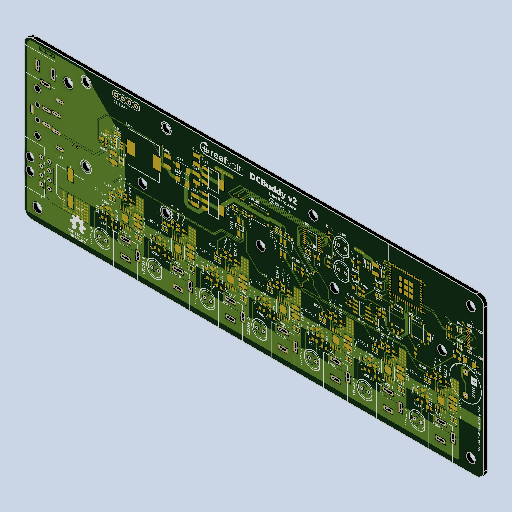
# Autodesk Inventor part: dcbuddy_v2_BOARD
Saved by Autodesk Inventor 2024.3 (Build 283343000, 343)
## iProperties
Created: 2024-05-05
Part Number: dcbuddy_v2_BOARD
Material: Generic
Document SubType Name: Modeling
Designer: atrus
Density: 1 g/cm^3
Appearance: BoardColor
Author: atrus
Autodesk Inventor part; units mm, degrees
ref_plane "YZ Plane" through (0, 0, 0) normal (1, 0, 0) x (0, 1, 0)
ref_plane "XZ Plane" through (0, 0, 0) normal (0, 1, 0) x (-1, 0, 0)
ref_plane "BoardFrontPlane" through (0, 0, 0) normal (0, 0, 1) x (1, 0, 0)
sketch "Sketch1" plane through (0, 0, 0) normal (0, 0, 1) x (1, 0, 0)
  arc A0 (36, 33) -> (39, 30) centre (39, 33) ccw
  line L0 (39, 30) -> (208, 30)
  arc A1 (208, 30) -> (211, 33) centre (208, 33) ccw
  line L1 (211, 33) -> (211, 87)
  arc A2 (211, 87) -> (208, 90) centre (208, 87) ccw
  line L2 (208, 90) -> (39, 90)
  arc A3 (39, 90) -> (36, 87) centre (39, 87) ccw
  line L3 (36, 87) -> (36, 33)
  constraints: 8 end point, 8 point on circle, 4 centre point
extrude "BoardOutline" add sketch "Sketch1" along normal blind 1.4202
sketch "Sketch19" plane through (0, 0, 1.4202) normal (0, 0, 1) x (1, 0, 0)
  point P0 (158.24, 80)
hole "LED301-C" at (158.24, 80, 1.4202) direction (0, 0, -1) diameter 0.8128 end through all
sketch "Sketch20" plane through (0, 0, 1.4202) normal (0, 0, 1) x (1, 0, 0)
  point P0 (155.7, 80)
hole "LED301-A" at (155.7, 80, 1.4202) direction (0, 0, -1) diameter 0.8128 end through all
sketch "Sketch21" plane through (0, 0, 1.4202) normal (0, 0, 1) x (1, 0, 0)
  point P0 (158.24, 72)
hole "LED300-C" at (158.24, 72, 1.4202) direction (0, 0, -1) diameter 0.8128 end through all
sketch "Sketch22" plane through (0, 0, 1.4202) normal (0, 0, 1) x (1, 0, 0)
  point P0 (155.7, 72)
hole "LED300-A" at (155.7, 72, 1.4202) direction (0, 0, -1) diameter 0.8128 end through all
sketch "Sketch23" plane through (0, 0, 1.4202) normal (0, 0, 1) x (1, 0, 0)
  point P0 (187.04, 37.25)
hole "LED200_CH7-C" at (187.04, 37.25, 1.4202) direction (0, 0, -1) diameter 0.8128 end through all
sketch "Sketch24" plane through (0, 0, 1.4202) normal (0, 0, 1) x (1, 0, 0)
  point P0 (184.5, 37.25)
hole "LED200_CH7-A" at (184.5, 37.25, 1.4202) direction (0, 0, -1) diameter 0.8128 end through all
sketch "Sketch25" plane through (0, 0, 1.4202) normal (0, 0, 1) x (1, 0, 0)
  point P0 (167.04, 37.25)
hole "LED200_CH6-C" at (167.04, 37.25, 1.4202) direction (0, 0, -1) diameter 0.8128 end through all
sketch "Sketch26" plane through (0, 0, 1.4202) normal (0, 0, 1) x (1, 0, 0)
  point P0 (164.5, 37.25)
hole "LED200_CH6-A" at (164.5, 37.25, 1.4202) direction (0, 0, -1) diameter 0.8128 end through all
sketch "Sketch27" plane through (0, 0, 1.4202) normal (0, 0, 1) x (1, 0, 0)
  point P0 (147.04, 37.25)
hole "LED200_CH5-C" at (147.04, 37.25, 1.4202) direction (0, 0, -1) diameter 0.8128 end through all
sketch "Sketch28" plane through (0, 0, 1.4202) normal (0, 0, 1) x (1, 0, 0)
  point P0 (144.5, 37.25)
hole "LED200_CH5-A" at (144.5, 37.25, 1.4202) direction (0, 0, -1) diameter 0.8128 end through all
sketch "Sketch29" plane through (0, 0, 1.4202) normal (0, 0, 1) x (1, 0, 0)
  point P0 (127.04, 37.25)
hole "LED200_CH4-C" at (127.04, 37.25, 1.4202) direction (0, 0, -1) diameter 0.8128 end through all
sketch "Sketch30" plane through (0, 0, 1.4202) normal (0, 0, 1) x (1, 0, 0)
  point P0 (124.5, 37.25)
hole "LED200_CH4-A" at (124.5, 37.25, 1.4202) direction (0, 0, -1) diameter 0.8128 end through all
sketch "Sketch31" plane through (0, 0, 1.4202) normal (0, 0, 1) x (1, 0, 0)
  point P0 (107.04, 37.25)
hole "LED200_CH3-C" at (107.04, 37.25, 1.4202) direction (0, 0, -1) diameter 0.8128 end through all
sketch "Sketch32" plane through (0, 0, 1.4202) normal (0, 0, 1) x (1, 0, 0)
  point P0 (104.5, 37.25)
hole "LED200_CH3-A" at (104.5, 37.25, 1.4202) direction (0, 0, -1) diameter 0.8128 end through all
sketch "Sketch33" plane through (0, 0, 1.4202) normal (0, 0, 1) x (1, 0, 0)
  point P0 (87.04, 37.25)
hole "LED200_CH2-C" at (87.04, 37.25, 1.4202) direction (0, 0, -1) diameter 0.8128 end through all
sketch "Sketch34" plane through (0, 0, 1.4202) normal (0, 0, 1) x (1, 0, 0)
  point P0 (84.5, 37.25)
hole "LED200_CH2-A" at (84.5, 37.25, 1.4202) direction (0, 0, -1) diameter 0.8128 end through all
sketch "Sketch35" plane through (0, 0, 1.4202) normal (0, 0, 1) x (1, 0, 0)
  point P0 (67.04, 37.25)
hole "LED200_CH1-C" at (67.04, 37.25, 1.4202) direction (0, 0, -1) diameter 0.8128 end through all
sketch "Sketch36" plane through (0, 0, 1.4202) normal (0, 0, 1) x (1, 0, 0)
  point P0 (64.5, 37.25)
hole "LED200_CH1-A" at (64.5, 37.25, 1.4202) direction (0, 0, -1) diameter 0.8128 end through all
sketch "Sketch37" plane through (0, 0, 1.4202) normal (0, 0, 1) x (1, 0, 0)
  line L0 (45, 77.3) -> (43, 77.3) construction
  line L1 (45, 77.8) -> (43, 77.8)
  line L2 (43, 76.8) -> (45, 76.8)
  arc A0 (45, 76.8) -> (45, 77.8) centre (45, 77.3) ccw
  arc A1 (43, 77.8) -> (43, 76.8) centre (43, 77.3) ccw
  point P0 (44, 77.3)
  constraints: 8 end point, 4 point on circle, 4 tangent, 2 centre point, 1 midpoint, 1 parallel
extrude "J701-3" cut sketch "Sketch37" against normal through all
sketch "Sketch38" plane through (0, 0, 1.4202) normal (0, 0, 1) x (1, 0, 0)
  line L0 (41, 81) -> (41, 83) construction
  line L1 (41.5, 81) -> (41.5, 83)
  line L2 (40.5, 83) -> (40.5, 81)
  arc A0 (40.5, 81) -> (41.5, 81) centre (41, 81) ccw
  arc A1 (41.5, 83) -> (40.5, 83) centre (41, 83) ccw
  point P0 (41, 82)
  constraints: 8 end point, 4 point on circle, 4 tangent, 2 centre point, 1 midpoint, 1 parallel
extrude "J701-2" cut sketch "Sketch38" against normal through all
sketch "Sketch39" plane through (0, 0, 1.4202) normal (0, 0, 1) x (1, 0, 0)
  line L0 (47, 80.75) -> (47, 83.25) construction
  line L1 (47.5, 80.75) -> (47.5, 83.25)
  line L2 (46.5, 83.25) -> (46.5, 80.75)
  arc A0 (46.5, 80.75) -> (47.5, 80.75) centre (47, 80.75) ccw
  arc A1 (47.5, 83.25) -> (46.5, 83.25) centre (47, 83.25) ccw
  point P0 (47, 82)
  constraints: 8 end point, 4 point on circle, 4 tangent, 2 centre point, 1 midpoint, 1 parallel
extrude "J701-1" cut sketch "Sketch39" against normal through all
sketch "Sketch40" plane through (0, 0, 1.4202) normal (0, 0, 1) x (1, 0, 0)
  line L0 (199.2, 39.25) -> (199.2, 37.25) construction
  line L1 (198.7, 39.25) -> (198.7, 37.25)
  line L2 (199.7, 37.25) -> (199.7, 39.25)
  arc A0 (199.7, 39.25) -> (198.7, 39.25) centre (199.2, 39.25) ccw
  arc A1 (198.7, 37.25) -> (199.7, 37.25) centre (199.2, 37.25) ccw
  point P0 (199.2, 38.25)
  constraints: 8 end point, 4 point on circle, 4 tangent, 2 centre point, 1 midpoint, 1 parallel
extrude "J200_CH7-3" cut sketch "Sketch40" against normal through all
sketch "Sketch41" plane through (0, 0, 1.4202) normal (0, 0, 1) x (1, 0, 0)
  line L0 (195.5, 35.25) -> (193.5, 35.25) construction
  line L1 (195.5, 35.75) -> (193.5, 35.75)
  line L2 (193.5, 34.75) -> (195.5, 34.75)
  arc A0 (195.5, 34.75) -> (195.5, 35.75) centre (195.5, 35.25) ccw
  arc A1 (193.5, 35.75) -> (193.5, 34.75) centre (193.5, 35.25) ccw
  point P0 (194.5, 35.25)
  constraints: 8 end point, 4 point on circle, 4 tangent, 2 centre point, 1 midpoint, 1 parallel
extrude "J200_CH7-2" cut sketch "Sketch41" against normal through all
sketch "Sketch42" plane through (0, 0, 1.4202) normal (0, 0, 1) x (1, 0, 0)
  line L0 (195.75, 41.25) -> (193.25, 41.25) construction
  line L1 (195.75, 41.75) -> (193.25, 41.75)
  line L2 (193.25, 40.75) -> (195.75, 40.75)
  arc A0 (195.75, 40.75) -> (195.75, 41.75) centre (195.75, 41.25) ccw
  arc A1 (193.25, 41.75) -> (193.25, 40.75) centre (193.25, 41.25) ccw
  point P0 (194.5, 41.25)
  constraints: 8 end point, 4 point on circle, 4 tangent, 2 centre point, 1 midpoint, 1 parallel
extrude "J200_CH7-1" cut sketch "Sketch42" against normal through all
sketch "Sketch43" plane through (0, 0, 1.4202) normal (0, 0, 1) x (1, 0, 0)
  line L0 (179.2, 39.25) -> (179.2, 37.25) construction
  line L1 (178.7, 39.25) -> (178.7, 37.25)
  line L2 (179.7, 37.25) -> (179.7, 39.25)
  arc A0 (179.7, 39.25) -> (178.7, 39.25) centre (179.2, 39.25) ccw
  arc A1 (178.7, 37.25) -> (179.7, 37.25) centre (179.2, 37.25) ccw
  point P0 (179.2, 38.25)
  constraints: 8 end point, 4 point on circle, 4 tangent, 2 centre point, 1 midpoint, 1 parallel
extrude "J200_CH6-3" cut sketch "Sketch43" against normal through all
sketch "Sketch44" plane through (0, 0, 1.4202) normal (0, 0, 1) x (1, 0, 0)
  line L0 (175.5, 35.25) -> (173.5, 35.25) construction
  line L1 (175.5, 35.75) -> (173.5, 35.75)
  line L2 (173.5, 34.75) -> (175.5, 34.75)
  arc A0 (175.5, 34.75) -> (175.5, 35.75) centre (175.5, 35.25) ccw
  arc A1 (173.5, 35.75) -> (173.5, 34.75) centre (173.5, 35.25) ccw
  point P0 (174.5, 35.25)
  constraints: 8 end point, 4 point on circle, 4 tangent, 2 centre point, 1 midpoint, 1 parallel
extrude "J200_CH6-2" cut sketch "Sketch44" against normal through all
sketch "Sketch45" plane through (0, 0, 1.4202) normal (0, 0, 1) x (1, 0, 0)
  line L0 (175.75, 41.25) -> (173.25, 41.25) construction
  line L1 (175.75, 41.75) -> (173.25, 41.75)
  line L2 (173.25, 40.75) -> (175.75, 40.75)
  arc A0 (175.75, 40.75) -> (175.75, 41.75) centre (175.75, 41.25) ccw
  arc A1 (173.25, 41.75) -> (173.25, 40.75) centre (173.25, 41.25) ccw
  point P0 (174.5, 41.25)
  constraints: 8 end point, 4 point on circle, 4 tangent, 2 centre point, 1 midpoint, 1 parallel
extrude "J200_CH6-1" cut sketch "Sketch45" against normal through all
sketch "Sketch46" plane through (0, 0, 1.4202) normal (0, 0, 1) x (1, 0, 0)
  line L0 (159.2, 39.25) -> (159.2, 37.25) construction
  line L1 (158.7, 39.25) -> (158.7, 37.25)
  line L2 (159.7, 37.25) -> (159.7, 39.25)
  arc A0 (159.7, 39.25) -> (158.7, 39.25) centre (159.2, 39.25) ccw
  arc A1 (158.7, 37.25) -> (159.7, 37.25) centre (159.2, 37.25) ccw
  point P0 (159.2, 38.25)
  constraints: 8 end point, 4 point on circle, 4 tangent, 2 centre point, 1 midpoint, 1 parallel
extrude "J200_CH5-3" cut sketch "Sketch46" against normal through all
sketch "Sketch47" plane through (0, 0, 1.4202) normal (0, 0, 1) x (1, 0, 0)
  line L0 (155.5, 35.25) -> (153.5, 35.25) construction
  line L1 (155.5, 35.75) -> (153.5, 35.75)
  line L2 (153.5, 34.75) -> (155.5, 34.75)
  arc A0 (155.5, 34.75) -> (155.5, 35.75) centre (155.5, 35.25) ccw
  arc A1 (153.5, 35.75) -> (153.5, 34.75) centre (153.5, 35.25) ccw
  point P0 (154.5, 35.25)
  constraints: 8 end point, 4 point on circle, 4 tangent, 2 centre point, 1 midpoint, 1 parallel
extrude "J200_CH5-2" cut sketch "Sketch47" against normal through all
sketch "Sketch48" plane through (0, 0, 1.4202) normal (0, 0, 1) x (1, 0, 0)
  line L0 (155.75, 41.25) -> (153.25, 41.25) construction
  line L1 (155.75, 41.75) -> (153.25, 41.75)
  line L2 (153.25, 40.75) -> (155.75, 40.75)
  arc A0 (155.75, 40.75) -> (155.75, 41.75) centre (155.75, 41.25) ccw
  arc A1 (153.25, 41.75) -> (153.25, 40.75) centre (153.25, 41.25) ccw
  point P0 (154.5, 41.25)
  constraints: 8 end point, 4 point on circle, 4 tangent, 2 centre point, 1 midpoint, 1 parallel
extrude "J200_CH5-1" cut sketch "Sketch48" against normal through all
sketch "Sketch49" plane through (0, 0, 1.4202) normal (0, 0, 1) x (1, 0, 0)
  line L0 (139.2, 39.25) -> (139.2, 37.25) construction
  line L1 (138.7, 39.25) -> (138.7, 37.25)
  line L2 (139.7, 37.25) -> (139.7, 39.25)
  arc A0 (139.7, 39.25) -> (138.7, 39.25) centre (139.2, 39.25) ccw
  arc A1 (138.7, 37.25) -> (139.7, 37.25) centre (139.2, 37.25) ccw
  point P0 (139.2, 38.25)
  constraints: 8 end point, 4 point on circle, 4 tangent, 2 centre point, 1 midpoint, 1 parallel
extrude "J200_CH4-3" cut sketch "Sketch49" against normal through all
sketch "Sketch50" plane through (0, 0, 1.4202) normal (0, 0, 1) x (1, 0, 0)
  line L0 (135.5, 35.25) -> (133.5, 35.25) construction
  line L1 (135.5, 35.75) -> (133.5, 35.75)
  line L2 (133.5, 34.75) -> (135.5, 34.75)
  arc A0 (135.5, 34.75) -> (135.5, 35.75) centre (135.5, 35.25) ccw
  arc A1 (133.5, 35.75) -> (133.5, 34.75) centre (133.5, 35.25) ccw
  point P0 (134.5, 35.25)
  constraints: 8 end point, 4 point on circle, 4 tangent, 2 centre point, 1 midpoint, 1 parallel
extrude "J200_CH4-2" cut sketch "Sketch50" against normal through all
sketch "Sketch51" plane through (0, 0, 1.4202) normal (0, 0, 1) x (1, 0, 0)
  line L0 (135.75, 41.25) -> (133.25, 41.25) construction
  line L1 (135.75, 41.75) -> (133.25, 41.75)
  line L2 (133.25, 40.75) -> (135.75, 40.75)
  arc A0 (135.75, 40.75) -> (135.75, 41.75) centre (135.75, 41.25) ccw
  arc A1 (133.25, 41.75) -> (133.25, 40.75) centre (133.25, 41.25) ccw
  point P0 (134.5, 41.25)
  constraints: 8 end point, 4 point on circle, 4 tangent, 2 centre point, 1 midpoint, 1 parallel
extrude "J200_CH4-1" cut sketch "Sketch51" against normal through all
sketch "Sketch52" plane through (0, 0, 1.4202) normal (0, 0, 1) x (1, 0, 0)
  line L0 (119.2, 39.25) -> (119.2, 37.25) construction
  line L1 (118.7, 39.25) -> (118.7, 37.25)
  line L2 (119.7, 37.25) -> (119.7, 39.25)
  arc A0 (119.7, 39.25) -> (118.7, 39.25) centre (119.2, 39.25) ccw
  arc A1 (118.7, 37.25) -> (119.7, 37.25) centre (119.2, 37.25) ccw
  point P0 (119.2, 38.25)
  constraints: 8 end point, 4 point on circle, 4 tangent, 2 centre point, 1 midpoint, 1 parallel
extrude "J200_CH3-3" cut sketch "Sketch52" against normal through all
sketch "Sketch53" plane through (0, 0, 1.4202) normal (0, 0, 1) x (1, 0, 0)
  line L0 (115.5, 35.25) -> (113.5, 35.25) construction
  line L1 (115.5, 35.75) -> (113.5, 35.75)
  line L2 (113.5, 34.75) -> (115.5, 34.75)
  arc A0 (115.5, 34.75) -> (115.5, 35.75) centre (115.5, 35.25) ccw
  arc A1 (113.5, 35.75) -> (113.5, 34.75) centre (113.5, 35.25) ccw
  point P0 (114.5, 35.25)
  constraints: 8 end point, 4 point on circle, 4 tangent, 2 centre point, 1 midpoint, 1 parallel
extrude "J200_CH3-2" cut sketch "Sketch53" against normal through all
sketch "Sketch54" plane through (0, 0, 1.4202) normal (0, 0, 1) x (1, 0, 0)
  line L0 (115.75, 41.25) -> (113.25, 41.25) construction
  line L1 (115.75, 41.75) -> (113.25, 41.75)
  line L2 (113.25, 40.75) -> (115.75, 40.75)
  arc A0 (115.75, 40.75) -> (115.75, 41.75) centre (115.75, 41.25) ccw
  arc A1 (113.25, 41.75) -> (113.25, 40.75) centre (113.25, 41.25) ccw
  point P0 (114.5, 41.25)
  constraints: 8 end point, 4 point on circle, 4 tangent, 2 centre point, 1 midpoint, 1 parallel
extrude "J200_CH3-1" cut sketch "Sketch54" against normal through all
sketch "Sketch55" plane through (0, 0, 1.4202) normal (0, 0, 1) x (1, 0, 0)
  line L0 (99.2, 39.25) -> (99.2, 37.25) construction
  line L1 (98.7, 39.25) -> (98.7, 37.25)
  line L2 (99.7, 37.25) -> (99.7, 39.25)
  arc A0 (99.7, 39.25) -> (98.7, 39.25) centre (99.2, 39.25) ccw
  arc A1 (98.7, 37.25) -> (99.7, 37.25) centre (99.2, 37.25) ccw
  point P0 (99.2, 38.25)
  constraints: 8 end point, 4 point on circle, 4 tangent, 2 centre point, 1 midpoint, 1 parallel
extrude "J200_CH2-3" cut sketch "Sketch55" against normal through all
sketch "Sketch56" plane through (0, 0, 1.4202) normal (0, 0, 1) x (1, 0, 0)
  line L0 (95.5, 35.25) -> (93.5, 35.25) construction
  line L1 (95.5, 35.75) -> (93.5, 35.75)
  line L2 (93.5, 34.75) -> (95.5, 34.75)
  arc A0 (95.5, 34.75) -> (95.5, 35.75) centre (95.5, 35.25) ccw
  arc A1 (93.5, 35.75) -> (93.5, 34.75) centre (93.5, 35.25) ccw
  point P0 (94.5, 35.25)
  constraints: 8 end point, 4 point on circle, 4 tangent, 2 centre point, 1 midpoint, 1 parallel
extrude "J200_CH2-2" cut sketch "Sketch56" against normal through all
sketch "Sketch57" plane through (0, 0, 1.4202) normal (0, 0, 1) x (1, 0, 0)
  line L0 (95.75, 41.25) -> (93.25, 41.25) construction
  line L1 (95.75, 41.75) -> (93.25, 41.75)
  line L2 (93.25, 40.75) -> (95.75, 40.75)
  arc A0 (95.75, 40.75) -> (95.75, 41.75) centre (95.75, 41.25) ccw
  arc A1 (93.25, 41.75) -> (93.25, 40.75) centre (93.25, 41.25) ccw
  point P0 (94.5, 41.25)
  constraints: 8 end point, 4 point on circle, 4 tangent, 2 centre point, 1 midpoint, 1 parallel
extrude "J200_CH2-1" cut sketch "Sketch57" against normal through all
sketch "Sketch58" plane through (0, 0, 1.4202) normal (0, 0, 1) x (1, 0, 0)
  line L0 (79.2, 39.25) -> (79.2, 37.25) construction
  line L1 (78.7, 39.25) -> (78.7, 37.25)
  line L2 (79.7, 37.25) -> (79.7, 39.25)
  arc A0 (79.7, 39.25) -> (78.7, 39.25) centre (79.2, 39.25) ccw
  arc A1 (78.7, 37.25) -> (79.7, 37.25) centre (79.2, 37.25) ccw
  point P0 (79.2, 38.25)
  constraints: 8 end point, 4 point on circle, 4 tangent, 2 centre point, 1 midpoint, 1 parallel
extrude "J200_CH1-3" cut sketch "Sketch58" against normal through all
sketch "Sketch59" plane through (0, 0, 1.4202) normal (0, 0, 1) x (1, 0, 0)
  line L0 (75.5, 35.25) -> (73.5, 35.25) construction
  line L1 (75.5, 35.75) -> (73.5, 35.75)
  line L2 (73.5, 34.75) -> (75.5, 34.75)
  arc A0 (75.5, 34.75) -> (75.5, 35.75) centre (75.5, 35.25) ccw
  arc A1 (73.5, 35.75) -> (73.5, 34.75) centre (73.5, 35.25) ccw
  point P0 (74.5, 35.25)
  constraints: 8 end point, 4 point on circle, 4 tangent, 2 centre point, 1 midpoint, 1 parallel
extrude "J200_CH1-2" cut sketch "Sketch59" against normal through all
sketch "Sketch60" plane through (0, 0, 1.4202) normal (0, 0, 1) x (1, 0, 0)
  line L0 (75.75, 41.25) -> (73.25, 41.25) construction
  line L1 (75.75, 41.75) -> (73.25, 41.75)
  line L2 (73.25, 40.75) -> (75.75, 40.75)
  arc A0 (75.75, 40.75) -> (75.75, 41.75) centre (75.75, 41.25) ccw
  arc A1 (73.25, 41.75) -> (73.25, 40.75) centre (73.25, 41.25) ccw
  point P0 (74.5, 41.25)
  constraints: 8 end point, 4 point on circle, 4 tangent, 2 centre point, 1 midpoint, 1 parallel
extrude "J200_CH1-1" cut sketch "Sketch60" against normal through all
sketch "Sketch61" plane through (0, 0, 1.4202) normal (0, 0, 1) x (1, 0, 0)
  point P0 (41, 58.7)
hole "J700-_DVCFIAIY" at (41, 58.7, 1.4202) direction (0, 0, -1) diameter 2.2 end through all
sketch "Sketch62" plane through (0, 0, 1.4202) normal (0, 0, 1) x (1, 0, 0)
  point P0 (41, 74.3)
hole "J700-_ODLUWIDP" at (41, 74.3, 1.4202) direction (0, 0, -1) diameter 2.2 end through all
sketch "Sketch63" plane through (0, 0, 1.4202) normal (0, 0, 1) x (1, 0, 0)
  line L0 (49.1, 69.4) -> (47.2, 69.4) construction
  line L1 (49.1, 69.7) -> (47.2, 69.7)
  line L2 (47.2, 69.1) -> (49.1, 69.1)
  arc A0 (49.1, 69.1) -> (49.1, 69.7) centre (49.1, 69.4) ccw
  arc A1 (47.2, 69.7) -> (47.2, 69.1) centre (47.2, 69.4) ccw
  point P0 (48.15, 69.4)
  constraints: 8 end point, 4 point on circle, 4 tangent, 2 centre point, 1 midpoint, 1 parallel
extrude "J700-1" cut sketch "Sketch63" against normal through all
sketch "Sketch64" plane through (0, 0, 1.4202) normal (0, 0, 1) x (1, 0, 0)
  line L0 (49.1, 63.6) -> (47.2, 63.6) construction
  line L1 (49.1, 63.9) -> (47.2, 63.9)
  line L2 (47.2, 63.3) -> (49.1, 63.3)
  arc A0 (49.1, 63.3) -> (49.1, 63.9) centre (49.1, 63.6) ccw
  arc A1 (47.2, 63.9) -> (47.2, 63.3) centre (47.2, 63.6) ccw
  point P0 (48.15, 63.6)
  constraints: 8 end point, 4 point on circle, 4 tangent, 2 centre point, 1 midpoint, 1 parallel
extrude "J700-2" cut sketch "Sketch64" against normal through all
sketch "Sketch65" plane through (0, 0, 1.4202) normal (0, 0, 1) x (1, 0, 0)
  line L0 (45.45, 69) -> (43.55, 69) construction
  line L1 (45.45, 69.3) -> (43.55, 69.3)
  line L2 (43.55, 68.7) -> (45.45, 68.7)
  arc A0 (45.45, 68.7) -> (45.45, 69.3) centre (45.45, 69) ccw
  arc A1 (43.55, 69.3) -> (43.55, 68.7) centre (43.55, 69) ccw
  point P0 (44.5, 69)
  constraints: 8 end point, 4 point on circle, 4 tangent, 2 centre point, 1 midpoint, 1 parallel
extrude "J700-3" cut sketch "Sketch65" against normal through all
sketch "Sketch66" plane through (0, 0, 1.4202) normal (0, 0, 1) x (1, 0, 0)
  line L0 (45.45, 64) -> (43.55, 64) construction
  line L1 (45.45, 64.3) -> (43.55, 64.3)
  line L2 (43.55, 63.7) -> (45.45, 63.7)
  arc A0 (45.45, 63.7) -> (45.45, 64.3) centre (45.45, 64) ccw
  arc A1 (43.55, 64.3) -> (43.55, 63.7) centre (43.55, 64) ccw
  point P0 (44.5, 64)
  constraints: 8 end point, 4 point on circle, 4 tangent, 2 centre point, 1 midpoint, 1 parallel
extrude "J700-4" cut sketch "Sketch66" against normal through all
sketch "Sketch67" plane through (0, 0, 1.4202) normal (0, 0, 1) x (1, 0, 0)
  line L0 (39, 65.7) -> (39, 67.3) construction
  line L1 (39.3, 65.7) -> (39.3, 67.3)
  line L2 (38.7, 67.3) -> (38.7, 65.7)
  arc A0 (38.7, 65.7) -> (39.3, 65.7) centre (39, 65.7) ccw
  arc A1 (39.3, 67.3) -> (38.7, 67.3) centre (39, 67.3) ccw
  point P0 (39, 66.5)
  constraints: 8 end point, 4 point on circle, 4 tangent, 2 centre point, 1 midpoint, 1 parallel
extrude "J700-SHLD_TGMFWFKS" cut sketch "Sketch67" against normal through all
sketch "Sketch68" plane through (0, 0, 1.4202) normal (0, 0, 1) x (1, 0, 0)
  point P0 (41, 64)
hole "J700-_CQXHUJUR" at (41, 64, 1.4202) direction (0, 0, -1) diameter 1.7 end through all
sketch "Sketch69" plane through (0, 0, 1.4202) normal (0, 0, 1) x (1, 0, 0)
  point P0 (41, 69)
hole "J700-_QRLXWSOT" at (41, 69, 1.4202) direction (0, 0, -1) diameter 1.7 end through all
sketch "Sketch70" plane through (0, 0, 1.4202) normal (0, 0, 1) x (1, 0, 0)
  line L0 (50.3, 58.7) -> (48.7, 58.7) construction
  line L1 (50.3, 59) -> (48.7, 59)
  line L2 (48.7, 58.4) -> (50.3, 58.4)
  arc A0 (50.3, 58.4) -> (50.3, 59) centre (50.3, 58.7) ccw
  arc A1 (48.7, 59) -> (48.7, 58.4) centre (48.7, 58.7) ccw
  point P0 (49.5, 58.7)
  constraints: 8 end point, 4 point on circle, 4 tangent, 2 centre point, 1 midpoint, 1 parallel
extrude "J700-SHLD_YFNGGBLJ" cut sketch "Sketch70" against normal through all
sketch "Sketch71" plane through (0, 0, 1.4202) normal (0, 0, 1) x (1, 0, 0)
  line L0 (50.3, 74.3) -> (48.7, 74.3) construction
  line L1 (50.3, 74.6) -> (48.7, 74.6)
  line L2 (48.7, 74) -> (50.3, 74)
  arc A0 (50.3, 74) -> (50.3, 74.6) centre (50.3, 74.3) ccw
  arc A1 (48.7, 74.6) -> (48.7, 74) centre (48.7, 74.3) ccw
  point P0 (49.5, 74.3)
  constraints: 8 end point, 4 point on circle, 4 tangent, 2 centre point, 1 midpoint, 1 parallel
extrude "J700-SHLD_BTUHUDDQ" cut sketch "Sketch71" against normal through all
sketch "Sketch72" plane through (0, 0, 1.4202) normal (0, 0, 1) x (1, 0, 0)
  line L0 (206.12, 69.7014) -> (205.02, 69.7014) construction
  line L1 (206.12, 70.0014) -> (205.02, 70.0014)
  line L2 (205.02, 69.4014) -> (206.12, 69.4014)
  arc A0 (206.12, 69.4014) -> (206.12, 70.0014) centre (206.12, 69.7014) ccw
  arc A1 (205.02, 70.0014) -> (205.02, 69.4014) centre (205.02, 69.7014) ccw
  point P0 (205.57, 69.7014)
  constraints: 8 end point, 4 point on circle, 4 tangent, 2 centre point, 1 midpoint, 1 parallel
extrude "J500-SH1" cut sketch "Sketch72" against normal through all
sketch "Sketch73" plane through (0, 0, 1.4202) normal (0, 0, 1) x (1, 0, 0)
  line L0 (206.12, 78.3414) -> (205.02, 78.3414) construction
  line L1 (206.12, 78.6414) -> (205.02, 78.6414)
  line L2 (205.02, 78.0414) -> (206.12, 78.0414)
  arc A0 (206.12, 78.0414) -> (206.12, 78.6414) centre (206.12, 78.3414) ccw
  arc A1 (205.02, 78.6414) -> (205.02, 78.0414) centre (205.02, 78.3414) ccw
  point P0 (205.57, 78.3414)
  constraints: 8 end point, 4 point on circle, 4 tangent, 2 centre point, 1 midpoint, 1 parallel
extrude "J500-SH2" cut sketch "Sketch73" against normal through all
sketch "Sketch74" plane through (0, 0, 1.4202) normal (0, 0, 1) x (1, 0, 0)
  line L0 (210.15, 69.7014) -> (209.35, 69.7014) construction
  line L1 (210.15, 70.0014) -> (209.35, 70.0014)
  line L2 (209.35, 69.4014) -> (210.15, 69.4014)
  arc A0 (210.15, 69.4014) -> (210.15, 70.0014) centre (210.15, 69.7014) ccw
  arc A1 (209.35, 70.0014) -> (209.35, 69.4014) centre (209.35, 69.7014) ccw
  point P0 (209.75, 69.7014)
  constraints: 8 end point, 4 point on circle, 4 tangent, 2 centre point, 1 midpoint, 1 parallel
extrude "J500-SH3" cut sketch "Sketch74" against normal through all
sketch "Sketch75" plane through (0, 0, 1.4202) normal (0, 0, 1) x (1, 0, 0)
  line L0 (210.15, 78.3414) -> (209.35, 78.3414) construction
  line L1 (210.15, 78.6414) -> (209.35, 78.6414)
  line L2 (209.35, 78.0414) -> (210.15, 78.0414)
  arc A0 (210.15, 78.0414) -> (210.15, 78.6414) centre (210.15, 78.3414) ccw
  arc A1 (209.35, 78.6414) -> (209.35, 78.0414) centre (209.35, 78.3414) ccw
  point P0 (209.75, 78.3414)
  constraints: 8 end point, 4 point on circle, 4 tangent, 2 centre point, 1 midpoint, 1 parallel
extrude "J500-SH4" cut sketch "Sketch75" against normal through all
sketch "Sketch76" plane through (0, 0, 1.4202) normal (0, 0, 1) x (1, 0, 0)
  point P0 (206.07, 76.9114)
hole "J500-_XJOSQWWH" at (206.07, 76.9114, 1.4202) direction (0, 0, -1) diameter 0.65 end through all
sketch "Sketch77" plane through (0, 0, 1.4202) normal (0, 0, 1) x (1, 0, 0)
  point P0 (206.07, 71.1314)
hole "J500-_OTGQXOCP" at (206.07, 71.1314, 1.4202) direction (0, 0, -1) diameter 0.65 end through all
sketch "Sketch78" plane through (0, 0, 1.4202) normal (0, 0, 1) x (1, 0, 0)
  point P0 (206, 85)
hole "Free-2_QOIIXSTY" at (206, 85, 1.4202) direction (0, 0, -1) diameter 3.4 end through all
sketch "Sketch79" plane through (0, 0, 1.4202) normal (0, 0, 1) x (1, 0, 0)
  point P0 (195, 65)
hole "Free-3" at (195, 65, 1.4202) direction (0, 0, -1) diameter 3.4 end through all
sketch "Sketch80" plane through (0, 0, 1.4202) normal (0, 0, 1) x (1, 0, 0)
  point P0 (41, 35)
hole "Free-8" at (41, 35, 1.4202) direction (0, 0, -1) diameter 3.4 end through all
sketch "Sketch83" plane through (0, 0, 1.4202) normal (0, 0, 1) x (1, 0, 0)
  point P0 (126, 65)
hole "Free-5" at (126, 65, 1.4202) direction (0, 0, -1) diameter 3.4 end through all
sketch "Sketch84" plane through (0, 0, 1.4202) normal (0, 0, 1) x (1, 0, 0)
  point P0 (154, 65)
hole "Free-4" at (154, 65, 1.4202) direction (0, 0, -1) diameter 3.4 end through all
sketch "Sketch85" plane through (0, 0, 1.4202) normal (0, 0, 1) x (1, 0, 0)
  point P0 (206, 35)
hole "Free-2_BIJDCKRQ" at (206, 35, 1.4202) direction (0, 0, -1) diameter 3.4 end through all
sketch "Sketch88" plane through (0, 0, 1.4202) normal (0, 0, 1) x (1, 0, 0)
  point P0 (38.18, 45.65)
hole "J702-_XCDHUICF" at (38.18, 45.65, 1.4202) direction (0, 0, -1) diameter 3 end through all
sketch "Sketch89" plane through (0, 0, 1.4202) normal (0, 0, 1) x (1, 0, 0)
  point P0 (38.18, 50.35)
hole "J702-_FYRNXHSV" at (38.18, 50.35, 1.4202) direction (0, 0, -1) diameter 3 end through all
sketch "Sketch90" plane through (0, 0, 1.4202) normal (0, 0, 1) x (1, 0, 0)
  point P0 (42.5, 52.51)
hole "J702-4" at (42.5, 52.51, 1.4202) direction (0, 0, -1) diameter 1.02 end through all
sketch "Sketch91" plane through (0, 0, 1.4202) normal (0, 0, 1) x (1, 0, 0)
  point P0 (42.5, 49.51)
hole "J702-3" at (42.5, 49.51, 1.4202) direction (0, 0, -1) diameter 1.02 end through all
sketch "Sketch92" plane through (0, 0, 1.4202) normal (0, 0, 1) x (1, 0, 0)
  point P0 (42.5, 46.51)
hole "J702-2" at (42.5, 46.51, 1.4202) direction (0, 0, -1) diameter 1.02 end through all
sketch "Sketch93" plane through (0, 0, 1.4202) normal (0, 0, 1) x (1, 0, 0)
  point P0 (42.5, 43.51)
hole "J702-1" at (42.5, 43.51, 1.4202) direction (0, 0, -1) diameter 1.02 end through all
sketch "Sketch94" plane through (0, 0, 1.4202) normal (0, 0, 1) x (1, 0, 0)
  point P0 (45.5, 43.51)
hole "J702-5" at (45.5, 43.51, 1.4202) direction (0, 0, -1) diameter 1.02 end through all
sketch "Sketch95" plane through (0, 0, 1.4202) normal (0, 0, 1) x (1, 0, 0)
  point P0 (45.5, 46.51)
hole "J702-6" at (45.5, 46.51, 1.4202) direction (0, 0, -1) diameter 1.02 end through all
sketch "Sketch96" plane through (0, 0, 1.4202) normal (0, 0, 1) x (1, 0, 0)
  point P0 (45.5, 49.51)
hole "J702-7" at (45.5, 49.51, 1.4202) direction (0, 0, -1) diameter 1.02 end through all
sketch "Sketch97" plane through (0, 0, 1.4202) normal (0, 0, 1) x (1, 0, 0)
  point P0 (45.5, 52.51)
hole "J702-8" at (45.5, 52.51, 1.4202) direction (0, 0, -1) diameter 1.02 end through all
sketch "Sketch98" plane through (0, 0, 1.4202) normal (0, 0, 1) x (1, 0, 0)
  point P0 (204, 54.7)
hole "SP300--" at (204, 54.7, 1.4202) direction (0, 0, -1) diameter 0.8 end through all
sketch "Sketch99" plane through (0, 0, 1.4202) normal (0, 0, 1) x (1, 0, 0)
  point P0 (204, 62.3)
hole "SP300-+" at (204, 62.3, 1.4202) direction (0, 0, -1) diameter 0.8 end through all
sketch "Sketch102" plane through (0, 0, 1.4202) normal (0, 0, 1) x (1, 0, 0)
  point P0 (59.52, 57.75)
hole "DISP800-_EDITXKCQ" at (59.52, 57.75, 1.4202) direction (0, 0, -1) diameter 3.048 end through all
sketch "Sketch103" plane through (0, 0, 1.4202) normal (0, 0, 1) x (1, 0, 0)
  point P0 (90, 57.75)
hole "DISP800-_RFTANGAA" at (90, 57.75, 1.4202) direction (0, 0, -1) diameter 3.048 end through all
sketch "Sketch104" plane through (0, 0, 1.4202) normal (0, 0, 1) x (1, 0, 0)
  point P0 (90, 85.69)
hole "DISP800-_UQJFIAXP" at (90, 85.69, 1.4202) direction (0, 0, -1) diameter 3.048 end through all
sketch "Sketch105" plane through (0, 0, 1.4202) normal (0, 0, 1) x (1, 0, 0)
  point P0 (78.57, 87.214)
hole "DISP800-4" at (78.57, 87.214, 1.4202) direction (0, 0, -1) diameter 1.016 end through all
sketch "Sketch106" plane through (0, 0, 1.4202) normal (0, 0, 1) x (1, 0, 0)
  point P0 (76.03, 87.214)
hole "DISP800-3" at (76.03, 87.214, 1.4202) direction (0, 0, -1) diameter 1.016 end through all
sketch "Sketch107" plane through (0, 0, 1.4202) normal (0, 0, 1) x (1, 0, 0)
  point P0 (73.49, 87.214)
hole "DISP800-2" at (73.49, 87.214, 1.4202) direction (0, 0, -1) diameter 1.016 end through all
sketch "Sketch108" plane through (0, 0, 1.4202) normal (0, 0, 1) x (1, 0, 0)
  point P0 (70.95, 87.214)
hole "DISP800-1" at (70.95, 87.214, 1.4202) direction (0, 0, -1) diameter 1.016 end through all
sketch "Sketch109" plane through (0, 0, 1.4202) normal (0, 0, 1) x (1, 0, 0)
  point P0 (59.52, 85.69)
hole "DISP800-_BEHFRQGU" at (59.52, 85.69, 1.4202) direction (0, 0, -1) diameter 3.048 end through all
sketch "Sketch110" plane through (0, 0, 1.4202) normal (0, 0, 1) x (1, 0, 0)
  point P0 (52.75, 82)
hole "Free-7" at (52.75, 82, 1.4202) direction (0, 0, -1) diameter 3.4 end through all
sketch "Sketch111" plane through (0, 0, 1.4202) normal (0, 0, 1) x (1, 0, 0)
  point P0 (81, 63)
hole "Free-6" at (81, 63, 1.4202) direction (0, 0, -1) diameter 3.4 end through all
sketch "Sketch112" plane through (0, 0, 1.4202) normal (0, 0, 1) x (1, 0, 0)
  point P0 (146, 85)
hole "Free-2_LYDOILJT" at (146, 85, 1.4202) direction (0, 0, -1) diameter 3.4 end through all
sketch "img_Top" plane through (0, 0, 1.4202) normal (0, 0, 1) x (1, 0, 0)
  line L0 (36, 90) -> (211, 90) construction
  line L1 (211, 90) -> (211, 30.0073) construction
  line L2 (211, 30.0073) -> (36, 30.0073) construction
  line L3 (36, 30.0073) -> (36, 90) construction
  constraints: 2 other
decal "Decal_Top"
sketch "img_Bottom" plane through (0, 0, -1.4202) normal (0, 0, -1) x (1, 0, 0)
  line L0 (36, -30) -> (211, -30) construction
  line L1 (211, -30) -> (211, -89.9927) construction
  line L2 (211, -89.9927) -> (36, -89.9927) construction
  line L3 (36, -89.9927) -> (36, -30) construction
  constraints: 2 other
decal "Decal_Bottom"
body "Solid1"
